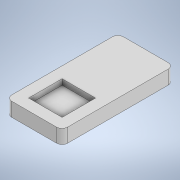
# Autodesk Inventor part: 維修門固定器
Saved by Autodesk Inventor 2021 (Build 250183000, 183)
## iProperties
Created: 2023-03-14
Part Number: 維修門固定器
Material: 一般
Document SubType Name: Modeling
Designer: brian
Density: 1 g/cm^3
Appearance: 預設
Author: brian
Autodesk Inventor part; units mm, degrees
ref_plane "YZ Plane" through (0, 0, 0) normal (1, 0, 0) x (0, 1, 0)
ref_plane "XZ Plane" through (0, 0, 0) normal (0, 1, 0) x (-1, 0, 0)
ref_plane "XY Plane" through (0, 0, 0) normal (0, 0, 1) x (1, 0, 0)
sketch "草圖1" plane through (0, 0, 0) normal (0, 1, 0) x (-1, 0, 0)
  line L0 (10, 20) -> (-10, 20)
  line L1 (-10, 20) -> (-10, -20)
  line L2 (-10, -20) -> (10, -20)
  line L3 (10, -20) -> (10, 20)
  line L4 (10, 20) -> (-10, -20) construction
  line L5 (-10, 20) -> (10, -20) construction
  point P0 (0, 0)
  dimension "d0" = 20
  dimension "d1" = 40
  constraints: 12 end point, 2 midpoint, 2 parallel, 1 horizontal, 1 perpendicular
  measures "d0" distance of L2.end L1.end
  measures "d1" distance of L1.end L0.end
extrude "擠出1" add sketch "草圖1" along normal mid plane 5
sketch "草圖2" plane through (0, -2.5, 0) normal (0, -1, 0) x (1, 0, 0)
  line L0 (-6, 4) -> (6, 4)
  line L1 (6, 4) -> (6, 16)
  line L2 (6, 16) -> (-6, 16)
  line L3 (-6, 16) -> (-6, 4)
  line L4 (-6, 4) -> (6, 16) construction
  line L5 (6, 4) -> (-6, 16) construction
  line L6 (10, 20) -> (-10, 20) projected
  point P0 (0, 0)
  point P1 (0, 10)
  point P2 (0, 10)
  dimension "d4" = 12
  dimension "d5" = 12
  dimension "d6" = 10
  constraints: 12 end point, 3 midpoint, 2 parallel, 1 horizontal, 1 perpendicular, 1 vertical alignment
  measures "d4" distance of L2.end L1.end
  measures "d5" distance of L1.end L0.end
  measures "d6" distance from line of L6 point (0, 10)
extrude "擠出2" cut sketch "草圖2" against normal blind 2
fillet "圓角1" radius 2 4 edges at (-10, 0, 20) (10, 0, 20) (10, 0, -20) (-10, 0, -20)
mirror "鏡射1" about plane through (0, 0, 0) normal (0, 1, 0) of "擠出2"
equation "\"d5\" = d4"
